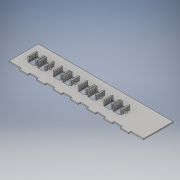
# Autodesk Inventor part: rear
Saved by Autodesk Inventor 2016 (Build 200138000, 138)
## iProperties
Created: 2015-08-26
Part Number: rear
Material: Generic
Document SubType Name: Modeling
Designer: gerthcm
Density: 1 g/cm^3
Appearance: Default
Author: gerthcm
Autodesk Inventor part; units mm, degrees
ref_plane "YZ Plane" through (0, 0, 0) normal (1, 0, 0) x (0, 1, 0)
ref_plane "XZ Plane" through (0, 0, 0) normal (0, 1, 0) x (-1, 0, 0)
ref_plane "XY Plane" through (0, 0, 0) normal (0, 0, 1) x (1, 0, 0)
sketch "Sketch1" plane through (0, 0, 0) normal (0, 1, 0) x (-1, 0, 0)
  line L0 (203.2, 31.75) -> (-203.2, 31.75)
  line L1 (-203.2, 31.75) -> (-203.2, -57.15)
  line L2 (-203.2, -57.15) -> (203.2, -57.15)
  line L3 (203.2, -57.15) -> (203.2, 31.75)
  point P0 (0, 0)
  point P1 (0, 0)
  dimension "d0" = 406.4
  dimension "d1" = 88.9
  constraints: 8 end point, 2 parallel, 1 horizontal, 1 perpendicular
  measures "d0" distance of L2.end L1.end
  measures "d1" distance of L1.end L0.end
extrude "Extrusion1" add sketch "Sketch1" along normal blind 3.175
sketch "Sketch3" plane through (0, 3.175, 0) normal (0, 1, 0) x (1, 0, 0)
  line L0 (-203.2, -31.75) -> (203.2, -31.75)
  line L1 (-165.1, -31.75) -> (-139.7, -31.75)
  line L2 (-139.7, -31.75) -> (-139.7, -38.1)
  line L3 (-139.7, -38.1) -> (-165.1, -38.1)
  line L4 (-165.1, -38.1) -> (-165.1, -31.75)
  line L5 (-114.3, -31.75) -> (-88.9, -31.75)
  line L6 (-88.9, -31.75) -> (-88.9, -38.1)
  line L7 (-88.9, -38.1) -> (-114.3, -38.1)
  line L8 (-114.3, -38.1) -> (-114.3, -31.75)
  line L9 (-63.5, -31.75) -> (-38.1, -31.75)
  line L10 (-38.1, -31.75) -> (-38.1, -38.1)
  line L11 (-38.1, -38.1) -> (-63.5, -38.1)
  line L12 (-63.5, -38.1) -> (-63.5, -31.75)
  line L13 (-12.7, -31.75) -> (12.7, -31.75)
  line L14 (12.7, -31.75) -> (12.7, -38.1)
  line L15 (12.7, -38.1) -> (-12.7, -38.1)
  line L16 (-12.7, -38.1) -> (-12.7, -31.75)
  line L17 (38.1, -31.75) -> (63.5, -31.75)
  line L18 (63.5, -31.75) -> (63.5, -38.1)
  line L19 (63.5, -38.1) -> (38.1, -38.1)
  line L20 (38.1, -38.1) -> (38.1, -31.75)
  line L21 (88.9, -31.75) -> (114.3, -31.75)
  line L22 (114.3, -31.75) -> (114.3, -38.1)
  line L23 (114.3, -38.1) -> (88.9, -38.1)
  line L24 (88.9, -38.1) -> (88.9, -31.75)
  line L25 (139.7, -31.75) -> (165.1, -31.75)
  line L26 (165.1, -31.75) -> (165.1, -38.1)
  line L27 (165.1, -38.1) -> (139.7, -38.1)
  line L28 (139.7, -38.1) -> (139.7, -31.75)
  point P0 (0, 0)
  point P1 (0, 0)
  dimension "d8" = 50.8
  constraints: 58 end point, 2 horizontal, 2 parallel, 1 collinear, 1 perpendicular, 1 point on line, 47 other
  measures "d8" distance of L1.start L5.start
extrude "Extrusion2" add sketch "Sketch3" against normal blind 3.175
sketch "Sketch4" plane through (-187.6003, 3.175, 12.867) normal (0, 1, 0) x (1, 0, 0)
  line L0 (15.875, 9.525) -> (34.925, 9.525)
  line L1 (34.925, 9.525) -> (34.925, 34.925)
  line L2 (34.925, 34.925) -> (15.875, 34.925)
  line L3 (15.875, 34.925) -> (15.875, 9.525)
  line L4 (44.45, 34.925) -> (63.5, 34.925)
  line L5 (63.5, 34.925) -> (63.5, 9.525)
  line L6 (63.5, 9.525) -> (44.45, 9.525)
  line L7 (44.45, 9.525) -> (44.45, 34.925)
  line L8 (92.075, 9.525) -> (111.125, 9.525)
  line L9 (111.125, 9.525) -> (111.125, 34.925)
  line L10 (111.125, 34.925) -> (92.075, 34.925)
  line L11 (92.075, 34.925) -> (92.075, 9.525)
  line L12 (120.65, 34.925) -> (139.7, 34.925)
  line L13 (139.7, 34.925) -> (139.7, 9.525)
  line L14 (139.7, 9.525) -> (120.65, 9.525)
  line L15 (120.65, 9.525) -> (120.65, 34.925)
  line L16 (168.275, 9.525) -> (187.325, 9.525)
  line L17 (187.325, 9.525) -> (187.325, 34.925)
  line L18 (187.325, 34.925) -> (168.275, 34.925)
  line L19 (168.275, 34.925) -> (168.275, 9.525)
  line L20 (196.85, 34.925) -> (215.9, 34.925)
  line L21 (215.9, 34.925) -> (215.9, 9.525)
  line L22 (215.9, 9.525) -> (196.85, 9.525)
  line L23 (196.85, 9.525) -> (196.85, 34.925)
  line L24 (244.475, 9.525) -> (263.525, 9.525)
  line L25 (263.525, 9.525) -> (263.525, 34.925)
  line L26 (263.525, 34.925) -> (244.475, 34.925)
  line L27 (244.475, 34.925) -> (244.475, 9.525)
  line L28 (273.05, 34.925) -> (292.1, 34.925)
  line L29 (292.1, 34.925) -> (292.1, 9.525)
  line L30 (292.1, 9.525) -> (273.05, 9.525)
  line L31 (273.05, 9.525) -> (273.05, 34.925)
  point P0 (160.3375, -5.08)
  dimension "d13" = 76.2
  constraints: 64 end point, 4 parallel, 4 point on line, 3 horizontal, 2 perpendicular, 1 collinear, 47 other
  measures "d13" distance of L0.start L8.start
extrude "Extrusion3" cut sketch "Sketch4" against normal blind 5
sketch "Sketch5" plane through (0, 3.175, 0) normal (0, 1, 0) x (1, 0, 0)
  line L0 (-171.45, -3.175) -> (-174.625, -3.175)
  line L1 (-174.625, -3.175) -> (-174.625, 22.225)
  line L2 (-174.625, 22.225) -> (-171.45, 22.225)
  line L3 (-171.45, 22.225) -> (-171.45, -3.175)
  line L4 (-152.4, 22.225) -> (-149.225, 22.225)
  line L5 (-149.225, 22.225) -> (-149.225, -3.175)
  line L6 (-149.225, -3.175) -> (-152.4, -3.175)
  line L7 (-152.4, -3.175) -> (-152.4, 22.225)
  line L8 (-124.1003, -3.342) -> (-143.1503, -3.342) projected
  line L9 (-143.1503, -3.342) -> (-146.05, -3.342)
  line L10 (-146.05, -3.342) -> (-146.05, 22.225)
  line L11 (-146.05, 22.225) -> (-143.1503, 22.225)
  line L12 (-143.1503, 22.225) -> (-143.1503, -3.342)
  line L13 (-124.1003, 22.225) -> (-120.65, 22.225)
  line L14 (-120.65, 22.225) -> (-120.65, -3.175)
  line L15 (-120.65, -3.175) -> (-124.1003, -3.175)
  line L16 (-124.1003, -3.175) -> (-124.1003, 22.225)
  line L17 (-73.025, 22.225) -> (-73.025, -3.175)
  line L18 (-76.2, 22.225) -> (-73.025, 22.225)
  line L19 (-76.2, -3.175) -> (-76.2, 22.225)
  line L20 (-95.25, 22.225) -> (-95.25, -3.175)
  line L21 (-98.425, -3.175) -> (-98.425, 22.225)
  line L22 (-98.425, 22.225) -> (-95.25, 22.225)
  line L23 (-95.25, -3.175) -> (-98.425, -3.175)
  line L24 (-73.025, -3.175) -> (-76.2, -3.175)
  line L25 (-69.85, -3.342) -> (-69.85, 22.225)
  line L26 (-69.85, 22.225) -> (-66.9503, 22.225)
  line L27 (-66.9503, -3.342) -> (-69.85, -3.342)
  line L28 (-66.9503, 22.225) -> (-66.9503, -3.342)
  line L29 (-44.45, -3.175) -> (-47.9003, -3.175)
  line L30 (-47.9003, -3.175) -> (-47.9003, 22.225)
  line L31 (-47.9003, 22.225) -> (-44.45, 22.225)
  line L32 (-44.45, 22.225) -> (-44.45, -3.175)
  line L33 (3.175, 22.225) -> (3.175, -3.175)
  line L34 (0, 22.225) -> (3.175, 22.225)
  line L35 (0, -3.175) -> (0, 22.225)
  line L36 (-19.05, 22.225) -> (-19.05, -3.175)
  line L37 (-22.225, -3.175) -> (-22.225, 22.225)
  line L38 (-22.225, 22.225) -> (-19.05, 22.225)
  line L39 (-19.05, -3.175) -> (-22.225, -3.175)
  line L40 (3.175, -3.175) -> (0, -3.175)
  line L41 (6.35, -3.342) -> (6.35, 22.225)
  line L42 (6.35, 22.225) -> (9.2497, 22.225)
  line L43 (9.2497, -3.342) -> (6.35, -3.342)
  line L44 (9.2497, 22.225) -> (9.2497, -3.342)
  line L45 (31.75, -3.175) -> (28.2997, -3.175)
  line L46 (28.2997, -3.175) -> (28.2997, 22.225)
  line L47 (28.2997, 22.225) -> (31.75, 22.225)
  line L48 (31.75, 22.225) -> (31.75, -3.175)
  line L49 (79.375, 22.225) -> (79.375, -3.175)
  line L50 (76.2, 22.225) -> (79.375, 22.225)
  line L51 (76.2, -3.175) -> (76.2, 22.225)
  line L52 (57.15, 22.225) -> (57.15, -3.175)
  line L53 (53.975, -3.175) -> (53.975, 22.225)
  line L54 (53.975, 22.225) -> (57.15, 22.225)
  line L55 (57.15, -3.175) -> (53.975, -3.175)
  line L56 (79.375, -3.175) -> (76.2, -3.175)
  line L57 (82.55, -3.342) -> (82.55, 22.225)
  line L58 (82.55, 22.225) -> (85.4497, 22.225)
  line L59 (85.4497, -3.342) -> (82.55, -3.342)
  line L60 (85.4497, 22.225) -> (85.4497, -3.342)
  line L61 (107.95, -3.175) -> (104.4997, -3.175)
  line L62 (104.4997, -3.175) -> (104.4997, 22.225)
  line L63 (104.4997, 22.225) -> (107.95, 22.225)
  line L64 (107.95, 22.225) -> (107.95, -3.175)
  point P0 (0, 0)
  dimension "d24" = 76.2
  constraints: 128 end point, 16 point on line, 8 parallel, 5 horizontal, 4 perpendicular, 1 collinear, 95 other
  measures "d24" distance of L0.start L20.end
extrude "Extrusion4" add sketch "Sketch5" along normal blind 12.7
sketch "Sketch6" plane through (-174.625, 3.175, -22.225) normal (-1, 0, 0) x (0, 0, 1)
  line L0 (19.05, 0) -> (15.875, 0)
  line L1 (15.875, 0) -> (15.875, 9.525)
  line L2 (15.875, 9.525) -> (19.05, 9.525)
  line L3 (19.05, 9.525) -> (19.05, 0)
  line L4 (9.525, 0) -> (6.35, 0)
  line L5 (6.35, 0) -> (6.35, 9.525)
  line L6 (6.35, 9.525) -> (9.525, 9.525)
  line L7 (9.525, 9.525) -> (9.525, 0)
  point P0 (22.225, -3.175)
  constraints: 16 end point, 4 parallel, 2 horizontal, 2 perpendicular
extrude "Extrusion5" cut sketch "Sketch6" against normal blind 406.4
chamfer "Chamfer1" distance 3.175 angle 45 8 edges at (-174.625, 3.175, -9.525) (-98.425, 3.175, -9.525) (-22.225, 3.175, -9.525) (53.975, 3.175, -9.525) (107.95, 3.175, -9.525) (31.75, 3.175, -9.525) (-44.45, 3.175, -9.525) (-120.65, 3.175, -9.525)
fillet "Fillet1" radius 3.175 8 edges at (-162.2003, 3.175, 3.342) (-133.6253, 3.175, 3.342) (-86.0003, 3.175, 3.342) (-57.4253, 3.175, 3.342) (-9.8003, 3.175, 3.342) (18.7747, 3.175, 3.342) (66.3997, 3.175, 3.342) (94.9747, 3.175, 3.342)
equation "\"d20\" = d21"
equation "\"d21\" = 5"
body "Solid1"
